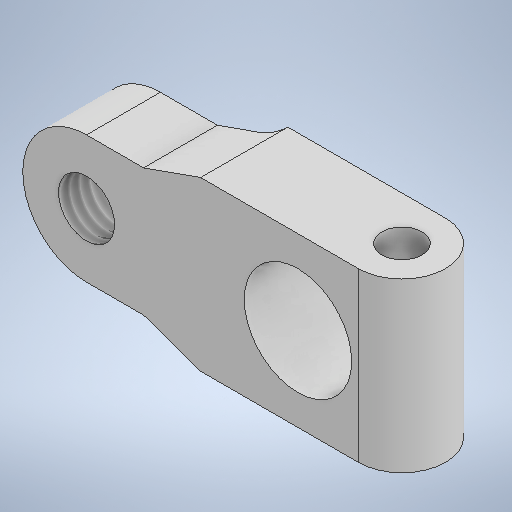
# Autodesk Inventor part: 2012
Saved by Autodesk Inventor 2025.1 (Build 291241000, 241)
## iProperties
Created: 2024-06-11
Part Number: 2012
Material: Generisch
Document SubType Name: Modeling
Designer: ffogue
Density: 1 g/cm^3
Appearance: Vorgabe
Author: ffogue
Autodesk Inventor part; units mm, degrees
ref_plane "YZ Plane" through (0, 0, 0) normal (1, 0, 0) x (0, 1, 0)
ref_plane "XZ Plane" through (0, 0, 0) normal (0, 1, 0) x (-1, 0, 0)
ref_plane "XY Plane" through (0, 0, 0) normal (0, 0, 1) x (1, 0, 0)
sketch "Skizze1" plane through (0, 0, 0) normal (0, 1, 0) x (-1, 0, 0)
  line L0 (0, 12.5) -> (0, -12.5)
  line L1 (0, -12.5) -> (30, -12.5)
  arc A0 (47, -9.5) -> (47, 9.5) centre (47, 0) ccw
  line L2 (47, 9.5) -> (38.5, 9.5)
  line L3 (38.5, 9.5) -> (30, 12.5)
  line L4 (30, 12.5) -> (0, 12.5)
  line L5 (0, 0) -> (47, 0) construction
  line L6 (30, -12.5) -> (38.5, -9.5)
  line L7 (38.5, -9.5) -> (47, -9.5)
  line L8 (30, 12.5) -> (30, -12.5)
  point P0 (56.5, 0)
  dimension "d0" = 90
  dimension "d1" = 25
  dimension "d2" = 30
  dimension "d3" = 47
  dimension "d5" = 8.5
  dimension "d6" = 18
  dimension "d9" = 30
  constraints: 18 end point, 3 horizontal, 3 point on circle, 3 vertical alignment, 1 centre point, 1 coincident, 1 horizontal alignment, 1 midpoint, 1 parallel, 1 symmetric about line, 1 tangent, 1 vertical
  measures "d0" angle of L0 L4
  measures "d1" distance of L0.start L0.end
  measures "d2" distance of L3.end L0.start
  measures "d3" distance from line of L0 L5.end
  measures "d5" horizontal distance of L2.end L3.end
  measures "d6" horizontal distance of point (56.5, 0) L2.end
  measures "d9" distance between parallel lines of L0 L8
extrude "Extrusion2" add sketch "Skizze1" along normal blind 13 contours L4 L8 L1 L0
extrude "Extrusion3" add sketch "Skizze1" along normal blind 11 contours L3 L2 A0 L7 L6 L8
fillet "Rundung1" radius 2 1 edges at (-30, 11, 0)
fillet "Rundung2" radius 6.5 2 edges at (0, 0, 0) (0, 13, 0)
sketch "Skizze2" plane through (-30, 0, -12.5) normal (0, 0, -1) x (-1, 0, 0)
  arc A0 (-23.5, 13) -> (-23.5, 0) centre (-23.5, 6.5) ccw projected
  point P0 (-30, 0)
  constraints: 1 coincident
hole "Bohrung1" at (-6.5, 6.5, -12.5) direction (0, 0, 1) diameter 6 depth 25
sketch "Skizze3" plane through (0, 11, 0) normal (0, 1, 0) x (1, 0, 0)
  arc A0 (-47, 9.5) -> (-47, -9.5) centre (-47, 0) ccw projected
  point P0 (0, 0)
  constraints: 1 coincident
hole "Bohrung2" at (-47, 11, 0) direction (0, -1, 0) diameter 8.376 depth 11 thread size "M10x1.5" class "6H" standard "ISO Metric profile"
sketch "Sketch4" plane through (0, 0, 0) normal (0, -1, 0) x (1, 0, 0)
  circle A0 centre (-15.5, 0) radius 8
  line L0 (-6.5, 12.5) -> (-6.5, -12.5) projected
  point P0 (0, 0)
  dimension "d30" = 16
  dimension "d33" = 9
  constraints: 1 centre point, 1 horizontal alignment
  measures "d30" diameter of A0
  measures "d33" distance from line of L0 A0.centre
extrude "Extrusion4" cut sketch "Sketch4" against normal up to surface (13 mm away)
